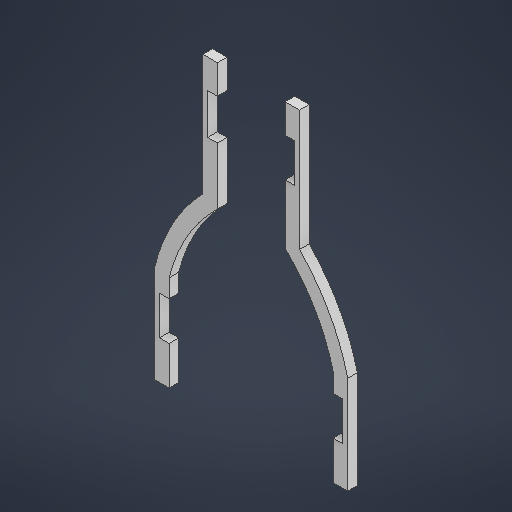
# Autodesk Inventor part: middlelsidewall
Saved by Autodesk Inventor 2026.2 (Build 302298000, 298)
## iProperties
Created: 2026-04-17
Part Number: middlelsidewall
Material: Generic
Document SubType Name: Modeling
Designer: danda
Density: 1 g/cm^3
Appearance: Default
Author: danda
Autodesk Inventor part; units mm, degrees
ref_plane "YZ Plane" through (0, 0, 0) normal (1, 0, 0) x (0, 1, 0)
ref_plane "XZ Plane" through (0, 0, 0) normal (0, 1, 0) x (-1, 0, 0)
ref_plane "XY Plane" through (0, 0, 0) normal (0, 0, 1) x (1, 0, 0)
sketch "Sketch2" plane through (0, 0, 0) normal (0, 0, 1) x (1, 0, 0)
  line L0 (372.3862, -40.1471) -> (372.3862, -100.1471)
  line L1 (337.3862, -40.1471) -> (337.3862, -100.1471)
  arc A0 (337.3862, -100.1471) -> (312.3862, -143.4484) centre (399.761, -165.0268) ccw
  line L2 (337.3862, -100.1471) -> (312.3862, -143.4484) construction
  line L3 (337.3862, -100.1471) -> (387.3862, -100.1471) construction
  line L4 (312.3862, -143.4484) -> (312.3862, -193.4484)
  arc A1 (397.248, -142.8964) -> (372.3862, -100.1471) centre (310.0113, -165.0268) ccw
  line L5 (397.248, -142.8964) -> (397.248, -192.8358)
  line L6 (347.3862, -193.4484) -> (347.3862, -148.2378)
  arc A2 (354.8862, -133.2267) -> (347.3862, -148.2378) centre (399.761, -165.0268) ccw
  arc A3 (362.248, -147.8127) -> (354.8862, -133.2267) centre (310.0113, -165.0268) ccw
  line L7 (362.248, -147.8127) -> (362.248, -192.8358)
  line L8 (304.8862, -192.8358) -> (304.8862, -142.5545)
  arc A4 (329.8862, -97.0286) -> (304.8862, -142.5545) centre (399.761, -165.0268) ccw
  line L9 (329.8862, -97.0286) -> (329.8862, -34.5346)
  line L10 (329.8862, -34.5346) -> (379.8862, -34.5346)
  line L11 (379.8862, -34.5346) -> (379.8862, -97.0286)
  arc A5 (404.8171, -142.2648) -> (379.8862, -97.0286) centre (310.0113, -165.0268) ccw
  line L12 (404.8171, -142.2648) -> (404.8171, -192.8358)
  line L13 (304.8862, -192.8358) -> (404.8171, -192.8358)
  line L14 (337.3862, -40.1471) -> (337.3862, -34.5346)
  line L15 (372.3862, -40.1471) -> (372.3862, -34.5346)
  line L16 (357.248, -192.8358) -> (357.248, -157.2921)
  line L17 (352.3862, -157.2921) -> (352.3862, -193.4484)
  line L18 (347.3862, -157.2921) -> (352.3862, -157.2921)
  line L19 (357.248, -157.2921) -> (362.248, -157.2921)
  line L20 (372.0272, -40.1471) -> (372.3862, -40.1471)
  line L21 (337.3862, -69.5346) -> (337.3862, -49.5346)
  line L22 (372.3862, -69.5346) -> (372.3862, -49.5346)
  line L23 (397.248, -172.8358) -> (397.248, -152.8358)
  line L24 (312.3862, -152.8358) -> (312.3862, -172.8358)
  line L25 (402.6367, -151.8358) -> (407.6367, -151.8358)
  line L26 (407.6367, -151.8358) -> (407.6367, -172.8358)
  line L27 (372.3862, -70.5346) -> (372.3862, -49.5346)
  line L28 (332.3862, -49.5346) -> (337.3862, -49.5346)
  line L29 (337.3862, -49.5346) -> (337.3862, -70.5346)
  line L30 (337.3862, -70.5346) -> (332.3862, -70.5346)
  line L31 (332.3862, -70.5346) -> (332.3862, -49.5346)
  line L32 (372.3862, -49.5346) -> (377.3866, -49.5346)
  line L33 (377.3866, -49.5346) -> (377.3866, -69.5346)
  line L34 (377.3866, -69.5346) -> (372.3862, -69.5346)
  line L35 (372.3862, -69.5346) -> (372.3862, -49.5346)
  line L36 (345.3862, -34.5346) -> (356.3862, -34.5346) construction
  line L37 (370.8862, -44.0609) -> (365.3862, -34.5346)
  line L38 (345.3862, -34.5346) -> (339.8862, -44.0609)
  line L39 (339.8862, -44.0609) -> (370.8862, -44.0609)
  line L40 (312.3862, -152.8358) -> (307.3862, -152.8358)
  line L41 (307.3862, -152.8358) -> (307.3862, -172.8358)
  line L42 (307.3862, -172.8358) -> (312.3862, -172.8358)
  line L43 (312.3862, -172.8358) -> (312.3862, -152.8358)
  line L44 (397.248, -152.8358) -> (402.248, -152.8358)
  line L45 (402.248, -152.8358) -> (402.248, -172.8358)
  line L46 (402.248, -172.8358) -> (397.248, -172.8358)
  line L47 (397.248, -172.8358) -> (397.248, -152.8358)
  point P0 (323.5989, -71.7026)
  point P1 (312.3862, -192.8358)
  dimension "d111" = 35
  dimension "d112" = 60
  dimension "d113" = 50
  dimension "d114" = 120
  dimension "d115" = 90
  dimension "d116" = 50
  dimension "d117" = 35
  dimension "d118" = 7.5
  dimension "d119" = 5
  dimension "d120" = 7.5
  dimension "d121" = 158.3013
  dimension "d122" = 0
  dimension "d123" = 21
  dimension "d124" = 5
  dimension "d125" = 21
  dimension "d126" = 15
  dimension "d127" = 2.5
  dimension "d128" = 15
  dimension "d129" = 5.0004
  dimension "d130" = 20
  dimension "d131" = 90
  dimension "d132" = 90
  dimension "d133" = 2.8196
  dimension "d134" = 10.3887
  dimension "d135" = 27.7505
  dimension "d136" = 30.2501
  dimension "d137" = 45.3887
  dimension "d138" = 55.2505
  dimension "d139" = 111.6887
  dimension "d140" = 51.6887
  dimension "d141" = 5.4563
  dimension "d142" = 84.0378
  dimension "d143" = 80.1333
  dimension "d144" = 9.571
  dimension "d145" = 1
  dimension "d146" = 102.3013
  dimension "d147" = 82.3013
  dimension "d148" = 81.3013
  dimension "d149" = 41.6125
  dimension "d150" = 41.6125
  dimension "d151" = 102.3013
  dimension "d152" = 82.3013
  dimension "d153" = 1
  dimension "d154" = 21
  dimension "d155" = 11
  dimension "d156" = 120
  dimension "d157" = 31
  dimension "d158" = 11
  dimension "d159" = 60
  dimension "d160" = 14.5
  dimension "d161" = 5
  dimension "d162" = 20
  dimension "d163" = 5
  dimension "d164" = 20
  dimension "d165" = 20
  dimension "d166" = 20
  constraints: 96 end point, 15 point on line, 14 parallel, 12 point on circle, 10 horizontal, 10 perpendicular, 6 centre point, 2 equal length, 2 vertical, 1 equal radius, 5 other
  measures "d111" distance of L1.start L20.end
  measures "d112" distance of L20.end L0.end
  measures "d113" distance of L1.end L4.start
  measures "d114" angle of L2 L3
  measures "d115" radius of A0
  measures "d116" distance of L4.start L4.end
  measures "d117" distance between parallel lines of L4 L6
  measures "d118" distance between parallel lines of L1 L9
  measures "d119" distance between parallel lines of L7 L16
  measures "d120" distance between parallel lines of L11 L0
  measures "d121" distance between parallel lines of L13 L10
  measures "d122" distance between parallel lines of L4 L24
  measures "d123" distance of L26.start L26.end
  measures "d124" distance of L29.end L30.end
  measures "d125" distance of L28.end L29.end
  measures "d126" distance between parallel lines of L10 L28
  measures "d127" distance between parallel lines of L9 L31
  measures "d128" distance between parallel lines of L10 L32
  measures "d129" distance of L33.end L35.start
  measures "d130" distance of L33.start L33.end
  measures "d131" angle of L25 L5
  measures "d132" angle of L27 L25
  measures "d133" distance between parallel lines of L12 L26
  measures "d134" distance between parallel lines of L23 L26
  measures "d135" distance between parallel lines of L26 L11
  measures "d136" distance between parallel lines of L26 L33
  measures "d137" distance between parallel lines of L26 L7
  measures "d138" distance between parallel lines of L17 L26
  measures "d139" distance between parallel lines of L25 L20
  measures "d140" distance between parallel lines of L25 L3
  measures "d141" distance between parallel lines of L25 L18
  measures "d142" distance from line of point (323.599, -71.703) L26
  measures "d143" distance from line of point (323.599, -71.703) L25
  measures "d144" distance from line of L12.start L25
  measures "d145" distance from line of L23.end L25
  measures "d146" distance from line of L22.end L25
  measures "d147" distance from line of L22.start L25
  measures "d148" distance from line of L27.start L25
  measures "d149" distance from line of L17.end L25
  measures "d150" distance from line of L6.start L25
  measures "d151" distance from line of L21.end L25
  measures "d152" distance from line of L21.start L25
  measures "d153" distance from line of L43.end L25
  measures "d154" distance from line of L24.end L25
  measures "d155" distance of L36.start L39.start
  measures "d156" angle of L38 L36
  measures "d157" distance of L39.start L37.start
  measures "d158" distance of L37.start L37.end
  measures "d159" angle of L39 L37
  measures "d160" distance of L11.start L37.end
  measures "d161" distance of L42.end L42.start
  measures "d162" distance of L42.start L41.start
  measures "d163" distance of L46.start L46.end
  measures "d164" distance of L45.start L46.start
  measures "d165" distance between parallel lines of L13 L46
  measures "d166" distance between parallel lines of L13 L42
extrude "Extrusion2" add sketch "Sketch2" along normal blind 5 contours L15 L10 L11 A5 L12 L13 L5 L46 L45 L44 A1 L0 L34 L33 L32 | L14 L1 L28 L31 L30 A0 L4 L40 L41 L42 L13 L8 A4 L9 L10
equation "\"d120\" = d118"
equation "\"d128\" = d126"
body "Solid2"
